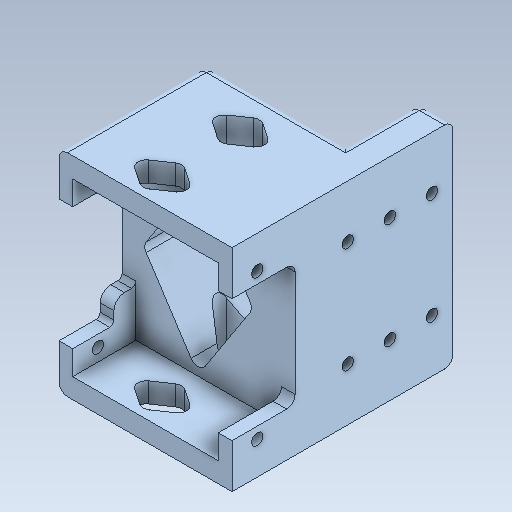
# Autodesk Inventor part: MotorCasing
Saved by Autodesk Inventor 2020 (Build 240168000, 168)
## iProperties
Created: 2019-10-13
Part Number: MotorCasing
Material: Generic
Document SubType Name: Modeling
Designer: ayad493
Density: 1 g/cm^3
Appearance: Light Steel Blue
Author: ayad493
Autodesk Inventor part; units mm, degrees
ref_plane "YZ Plane" through (0, 0, 0) normal (1, 0, 0) x (0, 1, 0)
ref_plane "XZ Plane" through (0, 0, 0) normal (0, 1, 0) x (-1, 0, 0)
ref_plane "XY Plane" through (0, 0, 0) normal (0, 0, 1) x (1, 0, 0)
sketch "Sketch1" plane through (0, 0, 0) normal (0, 0, 1) x (1, 0, 0)
  line L0 (0, 0) -> (44, 0)
  line L1 (0, 0) -> (-44, 0)
  line L2 (44, 0) -> (-44, 0)
  line L3 (44, 32.16) -> (44, -32.1598)
  line L4 (-44, -32.1598) -> (-44, 32.16)
  arc A0 (44, 32.1598) -> (-44, 32.1598) centre (0, 0) ccw
  arc A1 (-44, -32.1598) -> (44, -32.1598) centre (0, 0) ccw
  line L5 (-44, 32.16) -> (-43.9998, 32.16)
  line L6 (43.9998, 32.16) -> (44, 32.16)
  dimension "d1" = 44
  dimension "d2" = 44
  constraints: 14 end point, 6 point on circle, 5 horizontal, 2 centre point, 2 perpendicular, 2 point on line, 1 coincident, 1 parallel
  measures "d1" distance of L0.start L0.end
  measures "d2" distance of L0.start L1.end
extrude "Extrusion1" add sketch "Sketch1" along normal blind 5
sketch "Sketch2" plane through (0, 0, 5) normal (0, 0, 1) x (1, 0, 0)
  line L0 (-44, 32.1598) -> (-44, -32.1598) projected
  line L1 (-44, 0) -> (-44, -20.1)
  line L2 (-44, -20.1) -> (-44, 20.1)
  line L3 (-44, -20.1) -> (-40.5, -20.1)
  line L4 (-40.5, -20.1) -> (-40.5, 20.1)
  line L5 (-40.5, 20.1) -> (-44, 20.1)
  line L6 (-44, 20.1) -> (-44, -20.1)
  line L7 (-44, 0) -> (-6.4, 0)
  line L8 (-6.4, 0) -> (-6.4, 20.1)
  line L9 (-6.4, 20.1) -> (-2.9, 20.1)
  line L10 (-2.9, 20.1) -> (-2.9, -20.1)
  line L11 (-2.9, -20.1) -> (-6.4, -20.1)
  line L12 (-6.4, -20.1) -> (-6.4, 20.1)
  point P0 (0, 0)
  dimension "d6" = 20.1
  dimension "d7" = 40.2
  dimension "d8" = 3.5
  dimension "d9" = 37.6
  dimension "d10" = 20.1
  dimension "d11" = 3.5
  constraints: 24 end point, 4 parallel, 3 horizontal, 2 perpendicular, 2 point on line, 1 midpoint, 1 vertical
  measures "d6" distance of L1.start L1.end
  measures "d7" distance of L1.end L2.end
  measures "d8" distance of L5.end L4.end
  measures "d9" distance of L1.start L7.end
  measures "d10" distance of L7.end L8.end
  measures "d11" distance of L10.end L11.end
extrude "Extrusion2" add sketch "Sketch2" along normal blind 10
sketch "Sketch3" plane through (0, 0, 15) normal (0, 0, 1) x (1, 0, 0)
  line L0 (-40.5, 20.1) -> (-44, 20.1) projected
  line L1 (-44, 32.1598) -> (-44, -32.1598) projected
  line L2 (-40.5, 20.1) -> (-44, 20.1)
  line L3 (-44, 20.1) -> (-44, 14.6)
  line L4 (-44, 14.6) -> (-40.5, 14.6)
  line L5 (-40.5, 14.6) -> (-40.5, 20.1)
  line L6 (-2.9, 20.1) -> (-6.4, 20.1) projected
  line L7 (-6.4, 20.1) -> (-2.9, 20.1)
  line L8 (-2.9, 20.1) -> (-2.9, 14.6)
  line L9 (-2.9, 14.6) -> (-6.4, 14.6)
  line L10 (-6.4, 14.6) -> (-6.4, 20.1)
  line L11 (-40.5, 20.1) -> (-40.5, -20.1) projected
  line L12 (-40.5, -20.1) -> (-44, -20.1)
  line L13 (-44, -20.1) -> (-44, -14.6)
  line L14 (-44, -14.6) -> (-40.5, -14.6)
  line L15 (-40.5, -14.6) -> (-40.5, -20.1)
  line L16 (-6.4, -20.1) -> (-2.9, -20.1) projected
  line L17 (-6.4, 20.1) -> (-6.4, -20.1) projected
  line L18 (-2.9, -20.1) -> (-6.4, -20.1)
  line L19 (-6.4, -20.1) -> (-6.4, -14.6)
  line L20 (-6.4, -14.6) -> (-2.9, -14.6)
  line L21 (-2.9, -14.6) -> (-2.9, -20.1)
  point P0 (0, 0)
  dimension "d14" = 5.5
  dimension "d15" = 3.5
  dimension "d16" = 5.5
  dimension "d17" = 5.5
  constraints: 32 end point, 8 parallel, 4 horizontal, 4 perpendicular, 4 point on line
  measures "d14" distance of L3.end L2.end
  measures "d15" distance of L8.end L9.end
  measures "d16" distance of L7.end L8.end
  measures "d17" distance of L12.end L13.end
extrude "Extrusion3" add sketch "Sketch3" along normal blind 15 contours L5 L4 L1 L0 | L11 L12 L1 L14 | L8 L9 L10 L6 | L17 L20 L21 L16
sketch "Sketch4" plane through (0, 0, 5) normal (0, 0, 1) x (1, 0, 0)
  line L0 (-2.9, -20.1) -> (-6.4, -20.1) projected
  line L1 (-44, 20.1) -> (-40.5, 20.1) projected
  line L2 (-6.4, -20.1) -> (-40.5, -20.1)
  line L3 (-40.5, -20.1) -> (-40.5, 20.1)
  line L4 (-40.5, 20.1) -> (-6.4, 20.1)
  line L5 (-6.4, 20.1) -> (-6.4, -20.1)
  point P0 (0, 0)
  constraints: 8 end point, 2 parallel, 1 horizontal, 1 perpendicular
extrude "Extrusion4" add sketch "Sketch4" along normal blind 10
sketch "Sketch5" plane through (-44, -32.1598, 0) normal (-1, 0, 0) x (0, 0, 1)
  line L0 (15, 46.7598) -> (30, 46.7598) projected
  line L1 (15, 46.7598) -> (20.2, 46.7598)
  line L2 (20.2, 46.7598) -> (20.2, 43.8598)
  line L3 (17.7, 41.3598) -> (15, 41.3598)
  line L4 (15, 41.3598) -> (15, 46.7598)
  line L5 (15, 46.7598) -> (15, 17.5598) projected
  line L6 (15, 17.5598) -> (20.2, 17.5598)
  line L7 (20.2, 17.5598) -> (20.2, 20.4598)
  line L8 (17.7, 22.9598) -> (15, 22.9598)
  line L9 (15, 22.9598) -> (15, 17.5598)
  arc A0 (17.7, 41.3598) -> (20.2, 43.8598) centre (17.7, 43.8598) ccw
  arc A1 (20.2, 20.4598) -> (17.7, 22.9598) centre (17.7, 20.4598) ccw
  point P0 (0, 32.1598)
  point P1 (20.2, 41.3598)
  point P2 (20.2, 22.9598)
  dimension "d22" = 5.2
  dimension "d23" = 5.4
  dimension "d24" = 5.2
  dimension "d25" = 5.4
  dimension "d26" = 2.5
  constraints: 16 end point, 4 parallel, 4 point on circle, 4 point on line, 4 tangent, 2 centre point, 2 horizontal, 2 perpendicular, 1 equal radius
  measures "d22" distance of point (20.2, 41.36) L3.end
  measures "d23" distance of L1.end point (20.2, 41.36)
  measures "d24" distance of L8.end point (20.2, 22.96)
  measures "d25" distance of point (20.2, 22.96) L6.end
  measures "d26" radius of A0
extrude "Extrusion5" add sketch "Sketch5" against normal blind 3.5
fillet "Fillet1" radius 1 4 edges at (-42.25, 14.6, 20.2) (-42.25, 9.2, 15) (-42.25, -9.2, 15) (-42.25, -14.6, 20.2)
sketch "Sketch7" plane through (-44, -32.1598, 0) normal (-1, 0, 0) x (0, 0, 1)
  line L0 (5, 52.2598) -> (5, 12.0598) projected
  line L1 (5, 52.2598) -> (30, 52.2598)
  line L2 (30, 52.2598) -> (30, 57.2598)
  line L3 (30, 57.2598) -> (5, 57.2598)
  line L4 (5, 57.2598) -> (5, 52.2598)
  line L5 (15, 12.0598) -> (30, 12.0598) projected
  line L6 (5, 12.0598) -> (5, 0) projected
  line L7 (30, 12.0598) -> (5, 12.0598)
  line L8 (5, 12.0598) -> (5, 7.0598)
  line L9 (5, 7.0598) -> (30, 7.0598)
  line L10 (30, 7.0598) -> (30, 12.0598)
  point P0 (0, 32.1598)
  dimension "d34" = 5
  dimension "d35" = 5
  constraints: 16 end point, 4 parallel, 2 horizontal, 2 perpendicular, 1 point on line
  measures "d34" distance of L2.end L1.end
  measures "d35" distance of L8.end L7.end
extrude "Extrusion6" add sketch "Sketch7" against normal blind 41.1
sketch "Sketch8" plane through (-2.9, -14.6, 15) normal (1, 0, 0) x (0, 0, -1)
  line L0 (10, 39.7) -> (10, -10.5) projected
  line L1 (10, 14.6) -> (10, 47.6)
  line L2 (10, 47.6) -> (10, -18.4)
  line L3 (10, 47.6) -> (56, 47.6) construction
  line L4 (10, -18.4) -> (-36, -18.4)
  line L5 (10, -18.4) -> (56, -18.4) construction
  line L6 (10, -26.3) -> (-36, -26.3)
  line L7 (-36, -26.3) -> (-36, -10.5)
  line L8 (-36, -10.5) -> (10, -10.5)
  line L9 (10, -10.5) -> (10, -26.3)
  line L10 (10, -26.3) -> (-36, -10.5) construction
  line L11 (-36, -26.3) -> (10, -10.5) construction
  line L12 (-36, -26.3) -> (-31, -26.3)
  line L13 (-31, -26.3) -> (-31, -10.5)
  line L14 (-31, -10.5) -> (-36, -10.5)
  line L15 (-36, -10.5) -> (-36, -26.3)
  point P0 (15, 14.6)
  point P1 (-13, -18.4)
  point P2 (10, -10.5)
  dimension "d38" = 33
  dimension "d39" = 66
  dimension "d42" = 46
  dimension "d43" = 180
  dimension "d46" = 5
  constraints: 30 end point, 5 horizontal, 4 midpoint, 4 parallel, 2 collinear, 2 perpendicular, 2 point on line
  measures "d38" distance of L1.start L1.end
  measures "d39" distance of L1.end L2.end
  measures "d42" distance of L2.end L4.end
  measures "d43" angle of L4 L5
  measures "d46" distance of L14.end L13.end
extrude "Extrusion8" add sketch "Sketch8" along normal blind 6 contours L2 L4 L13 L8 | L9 L6 L13 L4
sketch "Sketch9" plane through (-2.9, -40.9, 46) normal (0, 0, 1) x (1, 0, 0)
  line L0 (0, 0) -> (0, 15.8) projected
  line L1 (0, 0) -> (11, 0)
  line L2 (11, 0) -> (11, 15.8)
  line L3 (7.5, 9.4) -> (4.5, 9.4)
  line L4 (4.5, 9.4) -> (4.5, 6.4)
  line L5 (4.5, 6.4) -> (7.5, 6.4)
  line L6 (7.5, 6.4) -> (7.5, 9.4)
  line L7 (6, 15.8) -> (6, 0) projected
  line L8 (7.5, 9.4) -> (4.5, 6.4) construction
  line L9 (4.5, 9.4) -> (7.5, 6.4) construction
  line L10 (12.5, 9.4) -> (9.5, 9.4)
  line L11 (9.5, 9.4) -> (9.5, 6.4)
  line L12 (9.5, 6.4) -> (12.5, 6.4)
  line L13 (12.5, 6.4) -> (12.5, 9.4)
  line L14 (12.5, 9.4) -> (9.5, 6.4) construction
  line L15 (9.5, 9.4) -> (12.5, 6.4) construction
  point P0 (2.9, 40.9)
  point P1 (6, 7.9)
  point P2 (11, 7.9)
  dimension "d50" = 11
  dimension "d51" = 3
  dimension "d52" = 3
  dimension "d53" = 3
  dimension "d54" = 3
  constraints: 28 end point, 6 midpoint, 4 parallel, 3 horizontal, 3 perpendicular
  measures "d50" distance of L0.start L1.end
  measures "d51" distance of L5.end L4.end
  measures "d52" distance of L4.end L3.end
  measures "d53" distance of L12.end L11.end
  measures "d54" distance of L11.end L10.end
extrude "Extrusion9" add sketch "Sketch9" against normal through all
sketch "Sketch10" plane through (-2.9, -40.9, 46) normal (0, 0, 1) x (1, 0, 0)
  line L0 (6, 0) -> (0, 0) projected
  line L1 (0, 0) -> (0, 15.8) projected
  line L2 (6, 0) -> (0, 0)
  line L3 (0, 0) -> (0, 15.8)
  line L4 (0, 15.8) -> (6, 15.8)
  line L5 (7.5, 6.4) -> (7.5, 9.4) projected
  line L6 (7.5, 9.4) -> (6, 9.4) projected
  line L7 (7.5, 6.4) -> (7.5, 9.4)
  line L8 (7.5, 9.4) -> (4.5, 9.4)
  line L9 (4.5, 9.4) -> (4.5, 6.4)
  line L10 (4.5, 6.4) -> (7.5, 6.4)
  line L11 (6, 15.8) -> (6, 9.4)
  line L12 (6, 6.4) -> (6, 0)
  point P0 (2.9, 40.9)
  dimension "d57" = 3
  constraints: 18 end point, 7 parallel, 2 midpoint, 2 perpendicular, 1 horizontal
  measures "d57" distance of L8.end L5.end
extrude "Extrusion10" cut sketch "Sketch10" against normal blind 41 contours L0 L1 L4 L11 L8 L9 L10 L12
sketch "Sketch11" plane through (0, 0, 5) normal (0, 0, 1) x (1, 0, 0)
  arc A0 (-44, -32.1598) -> (44, -32.1598) centre (0, 0) ccw projected
  line L0 (-44, -32.1598) -> (-44, -62.1598)
  line L1 (-44, -62.1598) -> (44, -62.1598)
  line L2 (44, -62.1598) -> (44, 63.4005)
  line L3 (44, 63.4005) -> (-44, 63.4005)
  line L4 (-44, 63.4005) -> (-44, -62.1598)
  line L5 (-2.9, -25.1) -> (-44, -25.1) projected
  line L6 (-44, 25.1) -> (-2.9, 25.1) projected
  line L7 (-2.9, -25.1) -> (-44, -25.1)
  line L8 (-44, -25.1) -> (-44, 25.1)
  line L9 (-44, 25.1) -> (-2.9, 25.1)
  line L10 (-2.9, 25.1) -> (-2.9, -25.1)
  line L11 (1.6, -34.5) -> (4.6, -34.5)
  line L12 (4.6, -34.5) -> (4.6, -31.5)
  line L13 (4.6, -31.5) -> (1.6, -31.5)
  line L14 (1.6, -31.5) -> (1.6, -34.5)
  line L15 (6.6, -34.5) -> (9.6, -34.5)
  line L16 (9.6, -34.5) -> (9.6, -31.5)
  line L17 (9.6, -31.5) -> (6.6, -31.5)
  line L18 (6.6, -31.5) -> (6.6, -34.5)
  point P0 (-44, -32.1598)
  dimension "d60" = 30
  constraints: 34 end point, 8 parallel, 4 horizontal, 4 perpendicular, 1 vertical
  measures "d60" distance of L0.start L0.end
extrude "Extrusion11" cut sketch "Sketch11" against normal blind 41 contours L4 L5 L10 L6 L3 L2 A0 | A0 L2 L1 L0
sketch "Sketch12" plane through (0, 0, 0) normal (0, 0, -1) x (-1, 0, 0)
  line L0 (44, 25.1) -> (2.9, 25.1) projected
  line L1 (2.9, -14.6) -> (2.9, -25.1) projected
  line L2 (2.9, 25.1) -> (2.9, -25.1)
  line L3 (2.9, -25.1) -> (-27.1, -25.1)
  line L4 (-27.1, -25.1) -> (-27.1, 25.1)
  line L5 (-27.1, 25.1) -> (2.9, 25.1)
  line L6 (2.9, 14.6) -> (2.9, 25.1) projected
  line L7 (2.9, 25.1) -> (44, 25.1)
  line L8 (44, 25.1) -> (44, -25.1)
  line L9 (44, -25.1) -> (2.9, -25.1)
  line L10 (2.9, -25.1) -> (2.9, 25.1)
  line L11 (2.9, 25.1) -> (2.9, -25.1) projected
  line L12 (2.9, 0) -> (2.9, -40)
  line L13 (2.9, 0) -> (2.9, 40)
  line L14 (7.9, -40) -> (-12.1, -40)
  line L15 (-12.1, -40) -> (2.9, -40)
  line L16 (2.9, -40) -> (2.9, 40)
  line L17 (2.9, 40) -> (-12.1, 40)
  line L18 (-12.1, 40) -> (-12.1, -40)
  point P0 (0, 0)
  point P1 (-12.1, 25.1)
  point P2 (-12.1, -25.1)
  dimension "d63" = 30
  dimension "d67" = 40
  dimension "d69" = 5
  dimension "d70" = 20
  dimension "d80" = 15
  constraints: 30 end point, 7 equal length, 3 perpendicular, 2 horizontal, 2 point on line, 1 midpoint, 1 vertical
  measures "d63" distance of L1.end L3.end
  measures "d67" distance of L12.start L13.end
  measures "d69" distance of L12.end L14.start
  measures "d70" distance of L14.start L14.end
  measures "d80" distance of L13.end L17.end
extrude "Extrusion13" add sketch "Sketch12" along normal blind 5
sketch "Sketch13" plane through (0, 0, -5) normal (0, 0, -1) x (-1, 0, 0)
  line L0 (2.9, 40) -> (-12.1, 40) projected
  line L1 (-12.1, -25.1) -> (-12.1, -40) projected
  line L2 (2.9, 40) -> (-12.1, 40)
  line L3 (-12.1, 40) -> (-12.1, -40)
  line L4 (-12.1, -40) -> (2.9, -40)
  line L5 (2.9, -40) -> (2.9, 40)
  point P0 (0, 0)
  constraints: 8 end point, 2 parallel, 1 horizontal, 1 perpendicular
extrude "Extrusion14" add sketch "Sketch13" along normal blind 10
sketch "Sketch14" plane through (12.1, 25.1, 0) normal (1, 0, 0) x (0, 0, -1)
  line L0 (15, 14.9) -> (15, -65.1) projected
  line L1 (15, -25.1) -> (15, -62.1)
  line L2 (15, -25.1) -> (15, 11.9)
  line L3 (15, -62.1) -> (23, -62.1)
  line L4 (15, 11.9) -> (23, 11.9)
  arc A0 (23, 3.9) -> (23, 19.9) centre (23, 11.9) ccw
  arc A1 (23, -70.1) -> (23, -54.1) centre (23, -62.1) ccw
  line L5 (23, 11.9) -> (15, 11.9)
  line L6 (15, 11.9) -> (15, -62.1)
  line L7 (15, -62.1) -> (23, -62.1)
  line L8 (23, -54.1) -> (23, 3.9)
  line L9 (15, -62.1) -> (0, -62.1)
  line L10 (0, -62.1) -> (0, -70.1)
  line L11 (0, -70.1) -> (23, -70.1)
  line L12 (23, 11.9) -> (0, 11.9)
  line L13 (0, 11.9) -> (0, 19.9)
  line L14 (0, 19.9) -> (23, 19.9)
  point P0 (0, -25.1)
  dimension "d75" = 37
  dimension "d76" = 37
  dimension "d77" = 8
  constraints: 28 end point, 4 horizontal, 4 parallel, 4 perpendicular, 4 point on circle, 4 point on line, 2 centre point, 2 coincident, 1 midpoint
  measures "d75" distance of L1.end L1.start
  measures "d76" distance of L2.end L1.start
  measures "d77" distance of L1.end L3.end
extrude "Extrusion15" add sketch "Sketch14" along normal blind 5 and the other way blind 15
sketch "Sketch15" plane through (12.1, -25.1, -5) normal (1, 0, 0) x (0, 0, -1)
  arc A0 (18, 54.1) -> (18, 70.1) centre (18, 62.1) ccw projected
  circle A1 centre (18, 62.1) radius 4
  arc A2 (18, -19.9) -> (18, -3.9) centre (18, -11.9) ccw projected
  circle A3 centre (18, -11.9) radius 4
  point P0 (-5, 25.1)
  dimension "d81" = 8
  constraints: 2 centre point, 2 coincident
  measures "d81" diameter of A1
extrude "Extrusion16" cut sketch "Sketch15" against normal through all
sketch "Sketch18" plane through (0, 0, -5) normal (0, 0, -1) x (-1, 0, 0)
  line L0 (-27.1, 25.1) -> (-27.1, -25.1) projected
  line L1 (-27.1, -25.1) -> (-12.1, -25.1) projected
  line L2 (-27.1, 25.1) -> (-12.1, 25.1)
  line L3 (-12.1, 25.1) -> (-12.1, -25.1)
  line L4 (-12.1, -25.1) -> (-27.1, -25.1)
  line L5 (-27.1, -25.1) -> (-27.1, 25.1)
  point P0 (0, 0)
  constraints: 8 end point, 2 parallel, 1 horizontal, 1 perpendicular
extrude "Extrusion19" cut sketch "Sketch18" against normal blind 5
sketch "Sketch19" plane through (12.1, -37, -15) normal (1, 0, 0) x (0, 0, -1)
  line L0 (0, 74) -> (-15, 74) projected
  line L1 (-15, -8) -> (-15, 11.9) projected
  line L2 (0, 74) -> (-15, 74)
  line L3 (-15, 74) -> (-15, -0.4336)
  line L4 (-15, -0.4336) -> (0, -0.4336)
  line L5 (0, -0.4336) -> (0, 74)
  point P0 (-15, 37)
  constraints: 8 end point, 2 parallel, 1 horizontal, 1 perpendicular, 1 point on line
extrude "Extrusion20" add sketch "Sketch19" along normal blind 5
sketch "Sketch20" plane through (-2.9, -25.1, -5) normal (-1, 0, 0) x (0, 0, 1)
  circle A0 centre (-18, -11.9) radius 4 projected
  circle A1 centre (-18, -11.9) radius 4
  circle A2 centre (-18, 62.1) radius 4 projected
  circle A3 centre (-18, 62.1) radius 4
  point P0 (5, 25.1)
  constraints: 2 centre point, 2 coincident
extrude "Extrusion21" cut sketch "Sketch20" against normal through all
sketch "Sketch21" plane through (17.1, 29, -23) normal (0, 0, -1) x (-1, 0, 0)
  line L0 (20, 0) -> (0, 0) projected
  line L1 (20, 0) -> (15, 0)
  line L2 (20, -58) -> (0, -58) projected
  line L3 (15, 0) -> (5, 0)
  line L4 (5, 0) -> (5, -58)
  line L5 (5, -58) -> (15, -58)
  line L6 (15, -58) -> (15, 0)
  line L7 (20, 16) -> (0, 16) projected
  line L8 (15, 0) -> (5, 0)
  line L9 (5, 0) -> (5, 16)
  line L10 (5, 16) -> (15, 16)
  line L11 (15, 16) -> (15, 0)
  line L12 (0, -74) -> (20, -74) projected
  line L13 (5, -58) -> (15, -58)
  line L14 (15, -58) -> (15, -74)
  line L15 (15, -74) -> (5, -74)
  line L16 (5, -74) -> (5, -58)
  point P0 (17.1, -29)
  dimension "d103" = 5
  dimension "d104" = 10
  constraints: 26 end point, 6 parallel, 6 point on line, 3 horizontal, 3 perpendicular
  measures "d103" distance of L0.start L1.end
  measures "d104" distance of L5.end L4.end
extrude "Extrusion22" cut sketch "Sketch21" along normal blind 8 and the other way blind 8
sketch "Sketch22" plane through (17.1, 29, -15) normal (0, 0, -1) x (-1, 0, 0)
  line L0 (5, -58) -> (0, -58) projected
  line L1 (20, -74) -> (15, -74) projected
  line L2 (5, -58) -> (15, -58)
  line L3 (15, -58) -> (15, -74)
  line L4 (15, -74) -> (5, -74)
  line L5 (5, -74) -> (5, -58)
  point P0 (17.1, -29)
  constraints: 8 end point, 2 parallel, 1 horizontal, 1 perpendicular
extrude "Extrusion23" cut sketch "Sketch22" against normal blind 15
sketch "Sketch23" plane through (17.1, 25.1, 0) normal (1, 0, 0) x (0, 0, -1)
  circle A0 centre (23, -62.1) radius 4 projected
  line L0 (23, -62.1) -> (13, -62.1)
  line L1 (13, -62.1) -> (13, -66.1)
  line L2 (13, -66.1) -> (13, -62.1)
  line L3 (13, -62.1) -> (13, -58.1)
  circle A1 centre (13, -66.1) radius 1.45
  circle A2 centre (13, -58.1) radius 1.45
  point P0 (0, -25.1)
  dimension "d111" = 10
  dimension "d112" = 4
  dimension "d113" = 4
  dimension "d118" = 2.9
  dimension "d119" = 2.9
  constraints: 8 end point, 2 centre point, 2 coincident, 1 collinear, 1 horizontal, 1 perpendicular, 1 point on line
  measures "d111" distance of L0.start L0.end
  measures "d112" distance of L0.end L1.end
  measures "d113" distance of L0.end L3.end
  measures "d118" diameter of A1
  measures "d119" diameter of A2
extrude "Extrusion25" cut sketch "Sketch23" against normal through all contours A1 | A2
sketch "Sketch24" plane through (1.6, -34.5, 46) normal (0, -1, 0) x (1, 0, 0)
  line L0 (8, 0) -> (8, -46) projected
  line L1 (5, 0) -> (5, -46) projected
  line L2 (8, -46) -> (5, -46)
  line L3 (5, -46) -> (5, 0)
  line L4 (5, 0) -> (8, 0)
  line L5 (8, 0) -> (8, -46)
  line L6 (3, 0) -> (3, -46) projected
  line L7 (0, 0) -> (3, 0)
  line L8 (3, 0) -> (3, -46)
  line L9 (3, -46) -> (0, -46)
  line L10 (0, -46) -> (0, 0)
  point P0 (-1.6, -46)
  constraints: 16 end point, 4 parallel, 2 horizontal, 2 perpendicular
extrude "Extrusion26" cut sketch "Sketch24" against normal blind 10
sketch "Sketch25" plane through (2.1, -29, -15) normal (0, -1, 0) x (1, 0, 0)
  line L0 (10, 0) -> (0, 0) projected
  line L1 (0, -8) -> (0, 15) projected
  line L2 (10, 0) -> (0, 0)
  line L3 (0, 0) -> (0, 5)
  line L4 (0, 5) -> (10, 5)
  line L5 (10, 5) -> (10, 0)
  point P0 (-2.1, 15)
  dimension "d124" = 5
  constraints: 8 end point, 2 parallel, 1 horizontal, 1 perpendicular, 1 point on line
  measures "d124" distance of L2.end L3.end
extrude "Extrusion27" cut sketch "Sketch25" against normal through all
chamfer "Chamfer1" distance 5 angle 45 1 edges at (-2.9, 0, -5)
chamfer "Chamfer2" distance 5 angle 45 1 edges at (-2.9, 0, 0)
sketch "Sketch26" plane through (17.1, 25.1, 0) normal (1, 0, 0) x (0, 0, -1)
  circle A0 centre (23, 11.9) radius 4 projected
  circle A1 centre (23, 11.9) radius 4
  circle A2 centre (23, -62.1) radius 4 projected
  circle A3 centre (23, -62.1) radius 4
  point P0 (0, -25.1)
  constraints: 2 centre point, 2 coincident
extrude "Extrusion28" add sketch "Sketch26" against normal blind 5
sketch "Sketch27" plane through (-2.9, -29, -23) normal (-1, 0, 0) x (0, 0, 1)
  circle A0 centre (0, 66) radius 4 projected
  circle A1 centre (0, 66) radius 4
  circle A2 centre (0, -8) radius 4 projected
  circle A3 centre (0, -8) radius 4
  point P0 (23, 29)
  constraints: 2 centre point, 2 coincident
extrude "Extrusion29" add sketch "Sketch27" against normal blind 5
sketch "Sketch28" plane through (17.1, 25.1, 0) normal (1, 0, 0) x (0, 0, -1)
  arc A0 (23, -70.1) -> (23, -54.1) centre (23, -62.1) ccw projected
  line L0 (23, -62.1) -> (31, -62.1)
  line L1 (23, -62.1) -> (24, -62.1)
  arc A1 (23, 3.9) -> (23, 19.9) centre (23, 11.9) ccw projected
  line L2 (23, 11.9) -> (31, 11.9)
  line L3 (23, 11.9) -> (24, 11.9)
  circle A2 centre (24, 11.9) radius 3
  circle A3 centre (24, -62.1) radius 3
  point P0 (0, -25.1)
  dimension "d138" = 1
  dimension "d139" = 1
  dimension "d140" = 6
  constraints: 8 end point, 2 centre point, 2 coincident, 2 horizontal, 2 point on circle, 2 point on line
  measures "d138" distance of L0.start L1.end
  measures "d139" distance of L2.start L3.end
  measures "d140" diameter of A3
extrude "Extrusion30" cut sketch "Sketch28" against normal through all
fillet "Fillet2" radius 2 2 edges at (-4.65, -14.6, 15) (-4.65, 14.6, 15)
sketch "Sketch29" plane through (-2.9, 14.6, 30) normal (1, 0, 0) x (0, 0, -1)
  line L0 (0, 0) -> (0, 10.5) projected
  line L1 (0, 0) -> (4, 0)
  line L2 (8.8, 0) -> (0, 0) projected
  line L3 (4, 0) -> (4, 2.7)
  line L4 (4, 2.7) -> (8, 2.7)
  circle A0 centre (6, 2.7) radius 1.35
  line L5 (13, -29.2) -> (0, -29.2) projected
  line L6 (0, -29.2) -> (4, -29.2)
  line L7 (4, -29.2) -> (4, -31.9)
  line L8 (15, -34.7) -> (0, -34.7) projected
  line L9 (4, -31.9) -> (6, -31.9)
  circle A1 centre (6, -31.9) radius 1.35
  line L10 (4, 2.7) -> (4, 5.5)
  line L11 (15, 5.5) -> (0, 5.5) projected
  point P0 (30, -14.6)
  dimension "d144" = 4
  dimension "d146" = 4
  dimension "d147" = 2.7
  dimension "d148" = 4
  dimension "d149" = 2.7
  dimension "d150" = 2
  dimension "d151" = 2.7
  dimension "d154" = 2.8
  constraints: 14 end point, 3 point on line, 2 centre point, 2 horizontal, 2 perpendicular, 1 coincident, 1 midpoint, 1 vertical
  measures "d144" distance of L0.start L1.end
  measures "d146" distance of L3.end L4.end
  measures "d147" diameter of A0
  measures "d148" distance of L5.end L6.end
  measures "d149" distance of L6.end L7.end
  measures "d150" distance of L7.end L9.end
  measures "d151" diameter of A1
  measures "d154" distance of L3.end L10.end
extrude "Extrusion31" cut sketch "Sketch29" against normal through all contours A0 L4 | L4 A0 | A1
sketch "Sketch30" plane through (0, 0, -5) normal (0, 0, -1) x (-1, 0, 0)
  line L0 (44, 25.1) -> (7.9, 25.1) projected
  line L1 (7.9, -25.1) -> (7.9, 25.1) projected
  line L2 (44, 25.1) -> (7.9, 25.1)
  line L3 (7.9, 25.1) -> (7.9, -25.1)
  line L4 (7.9, -25.1) -> (44, -25.1)
  line L5 (44, -25.1) -> (44, 25.1)
  line L6 (39, 20.1) -> (12.9, 20.1)
  line L7 (12.9, 20.1) -> (12.9, -20.1)
  line L8 (12.9, -20.1) -> (39, -20.1)
  line L9 (39, -20.1) -> (39, 20.1)
  line L10 (39, 0) -> (25.95, 20.1)
  line L11 (12.9, 0) -> (25.95, 20.1)
  line L12 (12.9, 0) -> (25.95, -20.1)
  line L13 (40.5, -20.1) -> (6.4, -20.1) projected
  line L14 (39, 0) -> (25.95, -20.1)
  point P0 (0, 0)
  dimension "d155" = 5
  constraints: 24 end point, 5 parallel, 3 midpoint, 2 perpendicular, 1 horizontal, 1 point on line, 3 other
  measures "d155" distance between parallel lines of L5 L9
extrude "Extrusion32" cut sketch "Sketch30" against normal through all contours L10 L14 L12 L11
fillet "Fillet3" radius 2 2 edges at (-25.95, -20.1, 5) (-25.95, 20.1, 5)
fillet "Fillet4" radius 2 2 edges at (-12.9, 0, 5) (-39, 0, 5)
sketch "Sketch31" plane through (-44, 25.1, 30) normal (0, 1, 0) x (1, 0, 0)
  line L0 (5.7071, 35) -> (16.3725, 35) projected
  line L1 (30.3929, 15) -> (30.7154, 15) projected
  line L2 (5.7071, 35) -> (30.3929, 35)
  line L3 (30.3929, 35) -> (30.3929, 15)
  line L4 (30.3929, 15) -> (5.7071, 15)
  line L5 (5.7071, 15) -> (5.7071, 35)
  line L6 (25.3929, 30) -> (10.7071, 30)
  line L7 (10.7071, 30) -> (10.7071, 20)
  line L8 (10.7071, 20) -> (25.3929, 20)
  line L9 (25.3929, 20) -> (25.3929, 30)
  line L10 (10.7071, 25) -> (18.05, 30)
  line L11 (10.7071, 25) -> (18.05, 20)
  line L12 (18.05, 20) -> (25.3929, 25)
  line L13 (18.05, 30) -> (25.3929, 25)
  line L14 (10.7071, 20) -> (10.7071, 11.5)
  line L15 (10.7071, 11.5) -> (25.3929, 11.5)
  line L16 (25.3929, 11.5) -> (25.3929, 1.5)
  line L17 (25.3929, 1.5) -> (10.7071, 1.5)
  line L18 (10.7071, 1.5) -> (10.7071, 11.5)
  line L19 (18.05, 11.5) -> (25.3929, 6.5)
  line L20 (25.3929, 6.5) -> (18.05, 1.5)
  line L21 (18.05, 11.5) -> (10.7071, 6.5)
  line L22 (18.05, 1.5) -> (10.7071, 6.5)
  point P0 (44, 30)
  dimension "d160" = 5
  dimension "d174" = 8.5
  dimension "d175" = 10
  constraints: 42 end point, 8 midpoint, 8 parallel, 3 perpendicular, 2 horizontal, 1 vertical, 3 other
  measures "d160" distance between parallel lines of L2 L6
  measures "d174" distance of L7.end L14.end
  measures "d175" distance of L15.end L16.end
extrude "Extrusion33" cut sketch "Sketch31" against normal through all contours L13 L12 L11 L10 | L19 L20 L22 L21
fillet "Fillet5" radius 2 16 edges at (-33.2929, 16.9451, 5) (-18.6071, 16.9451, 5) (-25.95, 21.7636, 0) (-25.95, 21.7636, 10) (-25.95, -21.7636, 10) (-25.95, -21.7636, 0) (-33.2929, -16.9451, 5) (-18.6071, -16.9451, 5) (-33.2929, 22.6, 23.5) (-25.95, 22.6, 28.5) (-18.6071, 22.6, 23.5) (-25.95, 22.6, 18.5) (-25.95, -22.6, 18.5) (-18.6071, -22.6, 23.5) (-25.95, -22.6, 28.5) (-33.2929, -22.6, 23.5)
fillet "Fillet6" radius 2 2 edges at (12.1, 8, -10) (2.1, 8, -10)
sketch "Sketch32" plane through (17.1, 25.1, 0) normal (1, 0, 0) x (0, 0, -1)
  arc A0 (23, 3.9) -> (23, 19.9) centre (23, 11.9) ccw projected
  line L0 (23, 11.9) -> (28.6569, 17.5569)
  line L1 (23, 11.9) -> (31, 11.9) construction
  arc A1 (23, -70.1) -> (23, -54.1) centre (23, -62.1) ccw projected
  line L2 (23, -62.1) -> (28.6569, -67.7569)
  circle A2 centre (28.6569, 17.5569) radius 2.5
  circle A3 centre (28.6569, -67.7569) radius 2.5
  point P0 (0, -25.1)
  point P1 (30.1267, -65.7346)
  point P2 (26.6346, -69.2267)
  point P3 (26.6346, 19.0267)
  point P4 (30.1267, 15.5346)
  dimension "d165" = 45
  dimension "d166" = 5
  dimension "d167" = 5
  constraints: 6 end point, 2 centre point, 2 coincident, 2 point on circle, 1 equal length, 1 horizontal
  measures "d165" angle of L1 L0
  measures "d166" diameter of A2
  measures "d167" diameter of A3
extrude "Extrusion34" add sketch "Sketch32" against normal up to surface (20 mm away) contours A0 A2 | A1 A3
sketch "Sketch33" plane through (17.1, -45, -23) normal (0, -1, 0) x (1, 0, 0)
  line L0 (-5, -3.6346) -> (-15, -3.6346) projected
  line L1 (-5, -3.6346) -> (-14.9875, -3.6346)
  line L2 (-14.9875, -3.6346) -> (-14.9875, -8.5279)
  line L3 (-14.9875, -8.5279) -> (-5, -8.5279)
  line L4 (-5, -8.5279) -> (-5, -3.6346)
  point P0 (-17.1, 23)
  constraints: 8 end point, 2 parallel, 1 horizontal, 1 perpendicular
extrude "Extrusion35" cut sketch "Sketch33" along normal blind 5 and the other way blind 100
fillet "Fillet7" radius 5 3 edges at (14.6, -45, 0) (-0.4, -45, 0) (7.1, 45, 0)
fillet "Fillet8" radius 5 4 edges at (14.6, -29, -23) (-0.4, -29, -23) (-0.4, 29, -23) (14.6, 29, -23)
sketch "Sketch35" plane through (-44, -25.1, 30) normal (0, -1, 0) x (1, 0, 0)
  line L0 (0, -35) -> (36.1, -35) projected
  line L1 (41.1, -30) -> (41.1, -40) projected
  line L2 (36.1, -35) -> (41.1, -35)
  line L3 (41.1, -35) -> (41.1, -40)
  line L4 (41.1, -40) -> (36.1, -40)
  line L5 (36.1, -40) -> (36.1, -35)
  line L6 (41.1, 0) -> (41.1, -25) projected
  line L7 (46.1, -30) -> (41.1, -25) projected
  line L8 (41.1, -25) -> (46.1, -25)
  line L9 (46.1, -25) -> (46.1, -30)
  line L10 (46.1, -30) -> (41.1, -30)
  line L11 (41.1, -30) -> (41.1, -25)
  point P0 (44, -30)
  constraints: 16 end point, 4 parallel, 2 horizontal, 2 perpendicular
extrude "Extrusion36" add sketch "Sketch35" against normal up to surface (50.2 mm away) contours L1 L4 L5 L2 | L7 L8 L9
sketch "Sketch36" plane through (12.1, 45, -23) normal (0, 1, 0) x (1, 0, 0)
  line L0 (-10, -28) -> (-15, -28) projected
  line L1 (0, 8) -> (5, 8) projected
  line L2 (-15, -28) -> (5, -28)
  line L3 (5, -28) -> (5, 8)
  line L4 (5, 8) -> (-15, 8)
  line L5 (-15, 8) -> (-15, -28)
  line L6 (5, 8) -> (-15, 8)
  line L7 (-15, 8) -> (-15, 13)
  line L8 (-15, 13) -> (5, 13)
  line L9 (5, 13) -> (5, 8)
  point P0 (-12.1, -23)
  dimension "d180" = 20
  dimension "d181" = 5
  constraints: 16 end point, 4 parallel, 2 horizontal, 2 perpendicular, 1 point on line
  measures "d180" distance of L0.end L2.end
  measures "d181" distance of L6.end L7.end
extrude "Extrusion37" cut sketch "Sketch36" along normal blind 10 and the other way blind 95
sketch "Sketch37" plane through (-7.9, -25.1, -10) normal (-1, 0, 0) x (0, 0, 1)
  line L0 (0, 0) -> (0, 50.2) projected
  line L1 (5, 50.2) -> (0, 50.2) projected
  line L2 (0, 50.2) -> (5, 50.2)
  line L3 (2.5, 50.2) -> (2.5, 0)
  line L4 (2.5, 0) -> (2.5, 25.1)
  line L5 (2.5, 50.2) -> (2.5, 25.1)
  line L6 (2.5, 25.1) -> (2.5, 0)
  line L7 (40, 0) -> (0, 0) projected
  circle A0 centre (2.5, 12.55) radius 1.35
  circle A1 centre (2.5, 37.65) radius 1.35
  point P0 (10, 25.1)
  dimension "d186" = 2.7
  dimension "d187" = 2.7
  constraints: 10 end point, 4 midpoint, 2 centre point, 2 collinear, 1 perpendicular, 1 vertical
  measures "d186" diameter of A0
  measures "d187" diameter of A1
extrude "Extrusion38" cut sketch "Sketch37" against normal through all contours A0 L3 | L3 A0 | A1 L3 | L3 A1
sketch "Sketch38" plane through (-2.9, 14.6, 30) normal (1, 0, 0) x (0, 0, -1)
  circle A0 centre (37.5, -2.05) radius 1.35 projected
  line L0 (37.5, -2.05) -> (27.5, -2.05)
  circle A1 centre (37.5, -27.15) radius 1.35 projected
  line L1 (27.5, -2.05) -> (37.5, -27.15)
  line L2 (37.5, -27.15) -> (27.5, -27.15)
  circle A2 centre (27.5, -2.05) radius 1.35
  circle A3 centre (27.5, -27.15) radius 1.35
  point P0 (30, -14.6)
  dimension "d190" = 10
  dimension "d191" = 10
  dimension "d192" = 2.7
  dimension "d193" = 2.7
  constraints: 6 end point, 2 centre point, 2 coincident, 1 horizontal, 1 parallel
  measures "d190" distance of L0.start L0.end
  measures "d191" distance of L1.end L2.end
  measures "d192" diameter of A2
  measures "d193" diameter of A3
extrude "Extrusion39" cut sketch "Sketch38" against normal blind 7 contours A2 L1 L0 | L0 L1 A2 | A3
sketch "Sketch39" plane through (0, 0, 15) normal (0, 0, 1) x (1, 0, 0)
  line L0 (-40.5, -20.1) -> (-6.4, -20.1) projected
  line L1 (-6.4, 20.1) -> (-6.4, 14.6) projected
  line L2 (-40.5, -20.1) -> (-6.4, -20.1)
  line L3 (-6.4, -20.1) -> (-6.4, 20.1)
  line L4 (-6.4, 20.1) -> (-40.5, 20.1)
  line L5 (-40.5, 20.1) -> (-40.5, -20.1)
  line L6 (-40.75, -20.35) -> (-6.15, -20.35)
  line L7 (-6.15, -20.35) -> (-6.15, 20.35)
  line L8 (-6.15, 20.35) -> (-40.75, 20.35)
  line L9 (-40.75, 20.35) -> (-40.75, -20.35)
  point P0 (0, 0)
  dimension "d196" = 0.25
  constraints: 16 end point, 4 parallel, 2 perpendicular, 1 horizontal, 3 other
  measures "d196" distance between parallel lines of L5 L9
extrude "Extrusion40" cut sketch "Sketch39" along normal up to surface (15 mm away)
fillet "Fillet9" radius 2 7 edges at (-5.4, -25.1, -10) (-5.4, 25.1, -10) (-25.95, -25.1, -5) (-44, 0, -5) (-25.95, 25.1, -5) (-44, 25.1, 12.5) (-44, -25.1, 12.5)
sketch "Sketch40" plane through (-2.9, 14.6, 30) normal (1, 0, 0) x (0, 0, -1)
  circle A0 centre (37.5, -2.05) radius 1.35 projected
  line L0 (37.5, -2.05) -> (52.5, -2.05)
  circle A1 centre (37.5, -27.15) radius 1.35 projected
  line L1 (37.5, -27.15) -> (52.5, -27.15)
  line L2 (0, -39.7) -> (38, -39.7) projected
  line L3 (37.5, -39.7) -> (52.5, -39.7)
  line L4 (52.5, -39.7) -> (52.5, -27.15)
  line L5 (52.5, -27.15) -> (37.5, -27.15)
  line L6 (37.5, -27.15) -> (37.5, -39.7)
  line L7 (52.5, -27.15) -> (37.5, -27.15)
  line L8 (37.5, -27.15) -> (37.5, -2.05)
  line L9 (37.5, -2.05) -> (52.5, -2.05)
  line L10 (52.5, -2.05) -> (52.5, -27.15)
  line L11 (0, 10.5) -> (38, 10.5) projected
  line L12 (37.5, -2.05) -> (37.5, 10.5)
  line L13 (37.5, 10.5) -> (52.5, 10.5)
  line L14 (52.5, 10.5) -> (52.5, -2.05)
  line L15 (52.5, -2.05) -> (37.5, -2.05)
  point P0 (30, -14.6)
  point P1 (37.5, -0.7)
  point P2 (37.5, -3.4)
  point P3 (37.5, -25.8)
  point P4 (38.85, -27.15)
  dimension "d200" = 15
  dimension "d201" = 15
  constraints: 28 end point, 6 parallel, 4 horizontal, 3 perpendicular, 2 point on line, 1 vertical
  measures "d200" distance of L0.start L0.end
  measures "d201" distance of L1.start L1.end
extrude "Extrusion41" add sketch "Sketch40" against normal blind 8 contours L0 L10 L1 A1 L8 A0 | A0 L12 L11 L13 L14 L0 | L4 L3 L2 L6 A1 L1 | A1 L6 L1
sketch "Sketch41" plane through (-2.9, -25.1, -22.5) normal (0, 0, -1) x (-1, 0, 0)
  line L0 (8, 0) -> (8, 12.55) projected
  line L1 (8, 0) -> (-0.0197, 0)
  line L2 (-0.0197, 0) -> (-0.0197, 50.2)
  line L3 (-0.0197, 50.2) -> (8, 50.2)
  line L4 (8, 50.2) -> (8, 0)
  point P0 (-2.9, 25.1)
  point P1 (8, 12.55)
  constraints: 8 end point, 2 parallel, 1 horizontal, 1 perpendicular
extrude "Extrusion42" add sketch "Sketch41" against normal blind 20
sketch "Sketch42" plane through (-2.8803, -25.1, -22.5) normal (1, 0, 0) x (0, 0, -1)
  circle A0 centre (-25, 37.65) radius 1.35 projected
  line L0 (-25, 37.65) -> (-15, 37.65)
  circle A1 centre (-25, 12.55) radius 1.35 projected
  line L1 (-25, 12.55) -> (-15, 12.55)
  line L2 (-25, 12.55) -> (-15, 12.55) construction
  line L3 (-15, 12.55) -> (-5, 12.55)
  line L4 (-15, 37.65) -> (-5, 37.65)
  circle A2 centre (-15, 37.65) radius 1.35
  circle A3 centre (-15, 12.55) radius 1.35
  circle A4 centre (-5, 12.55) radius 1.35
  circle A5 centre (-5, 37.65) radius 1.35
  point P0 (-22.5, 25.1)
  dimension "d206" = 10
  dimension "d207" = 10
  dimension "d208" = 0
  dimension "d209" = 10
  dimension "d210" = 10
  dimension "d211" = 2.7
  dimension "d212" = 2.7
  dimension "d213" = 2.7
  dimension "d214" = 2.7
  constraints: 10 end point, 4 centre point, 4 coincident, 4 horizontal, 1 collinear, 1 point on line
  measures "d206" distance of L0.start L0.end
  measures "d207" distance of L1.start L1.end
  measures "d208" distance between parallel lines of L1 L2
  measures "d209" distance of L1.end L3.end
  measures "d210" distance of L0.end L4.end
  measures "d211" diameter of A2
  measures "d212" diameter of A3
  measures "d213" diameter of A4
  measures "d214" diameter of A5
extrude "Extrusion43" cut sketch "Sketch42" against normal blind 20 contours A2 L4 L0 | L0 L4 A2 | A3 L3 L1 | L1 L3 A3 | A4 | A5
sketch "Sketch45" plane through (-2.9, -25.1, -2.5) normal (0, 0, 1) x (1, 0, 0)
  line L0 (0, 0) -> (0, 50.2) projected
  line L1 (0, 0) -> (0.0198, 0)
  line L2 (0.0198, 0) -> (0.0198, 50.2)
  line L3 (0.0198, 50.2) -> (0, 50.2)
  line L4 (0, 50.2) -> (0, 0)
  point P0 (2.9, 25.1)
  constraints: 8 end point, 2 parallel, 1 horizontal, 1 perpendicular
extrude "Extrusion44" cut sketch "Sketch45" against normal blind 20
fillet "Fillet10" radius 2 5 edges at (-10.9, 25.1, -12.75) (-10.9, 0, -22.5) (-10.9, -25.1, -12.75) (-6.9, 25.1, -22.5) (-6.9, -25.1, -22.5)
body "Solid1"
